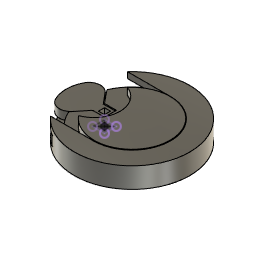
TotemMount (Autodesk Fusion 360 design; units mm, degrees)
Autodesk Fusion 360 part; units mm, degrees
sketch "Sketch1" plane through (0, 0, 0) normal (0, 0, 1) x (1, 0, 0)
  circle A0 centre (0, 0) radius 48
  dimension "d1" = 96
  constraint coincident A0.centre origin
  measures "d1" diameter of A0
extrude "Extrude1" add sketch "Sketch1" along normal blind 4 makes body 1
sketch "Sketch2" plane through (0, 0, 4) normal (0, 0, 1) x (-1, 0, 0)
  circle A0 centre (0, 0) radius 48
  line L0 (0, 0) -> (18, 0)
  line L1 (18, -4.925) -> (18, 4.925)
  line L2 (18, -4.925) -> (27.85, -4.925)
  line L3 (27.85, -4.925) -> (27.85, 4.925)
  line L4 (27.85, 4.925) -> (18, 4.925)
  circle A1 centre (0, 0) radius 40
  line L5 (0, -40) -> (50, -40)
  line L6 (0, 40) -> (50, 40)
  dimension "d4" = 18
  dimension "d5" = 9.85
  dimension "d6" = 8
  constraint coincident A0.centre L0.start
  constraint horizontal L0
  constraint vertical L1
  constraint midpoint L0.end L1
  constraint perpendicular L1 L2
  constraint equal L1 L2
  constraint perpendicular L2 L3
  constraint perpendicular L3 L4
  constraint concentric A0 A1
  constraint coincident A1 L5.start
  constraint tangent A1 L5
  constraint horizontal L5
  constraint coincident A1 L6.start
  constraint tangent A1 L6
  constraint horizontal L6
  measures "d4" distance of A0.centre L0.end
  measures "d5" distance of L1.start L2.end
  measures "d6" distance of A0 A1
extrude "Extrude2" cut sketch "Sketch2" against normal blind 30 contours L1 L2 L3 L4 bodies 1
extrude "Extrude3" add sketch "Sketch2" along normal blind 8 contours A0 A1 L5 L6 picked at (2.0777, 45.1772) bodies 1
sketch "Sketch3" plane through (0, 0, 12) normal (0, 0, 1) x (-1, 0, 0)
  arc A0 (0, 40) -> (0, -40) centre (0, 0) ccw
  line L0 (0, 40) -> (26.533, 40)
  arc A1 (26.533, 40) -> (26.533, -40) centre (0, 0) ccw
  line L1 (26.533, -40) -> (0, -40)
  circle A2 centre (0, 0) radius 32
  circle A3 centre (0, 0) radius 40
  line L2 (0, -32) -> (50, -32)
  line L3 (0, 32) -> (50.0906, 32)
  circle A4 centre (0, 0) radius 48
  circle A5 centre (0, 0) radius 48
  dimension "d11" = 8
  constraint coincident A0.centre A1.centre
  constraint coincident A2 L2.start
  constraint horizontal L2
  constraint coincident A2 L3.start
  constraint horizontal L3
  constraint collinear A0.start A0.end L2.start
  constraint collinear A0.start L2.start L3.start
  constraint concentric A2 A4
  constraint equal A4 A5
  measures "d11" distance of A2 A3
extrude "Extrude4" add sketch "Sketch3" along normal blind 5 contours A0 A2 A3 L2 L3 | A0 L0 A1 L1 A3 A4 A5 | L0 A3 L3 A4 A5 | L1 A3 L2 A4 A5 bodies 1
sketch "Sketch4" plane through (0, 0, 4) normal (0, 0, 1) x (-1, 0, 0)
  circle A0 centre (0, 0) radius 39.8
  circle A1 centre (0, 0) radius 40
  dimension "d14" = 0.2
  constraint coincident A0.centre A1.centre
  measures "d14" distance of A0 A1
extrude "Extrude5" add sketch "Sketch2" along normal blind 7.6 separate body contours A1 makes body 2
sketch "Sketch5" plane through (0, 0, 11.6) normal (0, 0, 1) x (-1, 0, 0)
  line L0 (27.85, -4.925) -> (18, -4.925)
  line L1 (18, -4.925) -> (18, 4.925)
  line L2 (18, 4.925) -> (27.85, 4.925)
  line L3 (27.85, 4.925) -> (27.85, -4.925)
  circle A0 centre (0, 0) radius 31.6
  arc A1 (0, 32) -> (0, -32) centre (0, 0) ccw
  circle A2 centre (31.6, 0) radius 21.6
  circle A3 centre (0, 0) radius 40
  dimension "d17" = 0.4
  dimension "d18" = 43.2
  constraint coincident A0 A2.centre
  measures "d17" distance of A0 A1
  measures "d18" diameter of A2
extrude "Extrude6" add sketch "Sketch5" along normal blind 5.7 contours A0 A2 picked at (-17.657, 0.5171) bodies 2
sketch "Sketch6" plane through (0, 0, 11.6) normal (0, 0, 1) x (-1, 0, 0)
  arc A0 (24.2177, 20.2993) -> (24.2177, -20.2993) centre (31.6, 0) ccw
  arc A1 (24.2177, 20.2993) -> (24.2177, -20.2993) centre (0, 0) ccw
  line L0 (27.85, -4.925) -> (18, -4.925)
  line L1 (18, -4.925) -> (18, 4.925)
  line L2 (18, 4.925) -> (27.85, 4.925)
  line L3 (27.85, 4.925) -> (27.85, -4.925)
  line L4 (27.85, -4.925) -> (36.7179, -15.868)
  line L5 (27.85, 4.925) -> (36.7179, 15.868)
  circle A2 centre (0, 0) radius 40
  constraint coincident L0.start L3.end
  constraint coincident L4.end A2
  constraint coincident L2.end L3.start
  constraint coincident L5.end A2
extrude "Extrude8" cut sketch "Sketch6" against normal blind 10 contours L3 L4 L5 A2 bodies 2
sketch "Sketch7" plane through (0, 0, 0) normal (0, 0, 1) x (1, 0, 0)
  line L0 (-27.55, 4.625) -> (-18.3, 4.625)
  line L1 (-18.3, 4.625) -> (-18.3, -4.625)
  line L2 (-18.3, -4.625) -> (-27.55, -4.625)
  line L3 (-27.55, -4.625) -> (-27.55, 4.625)
  line L4 (-27.55, 4.625) -> (-18.3, -4.625) construction
  line L5 (-18.3, 4.625) -> (-27.55, -4.625) construction
  line L6 (-18, 4.925) -> (-27.85, 4.925)
  line L7 (-27.85, -4.925) -> (-18, -4.925)
  line L8 (-18, 4.925) -> (-18, -4.925)
  line L9 (-25.425, 2.5) -> (-20.425, 2.5)
  line L10 (-20.425, 2.5) -> (-20.425, -2.5)
  line L11 (-20.425, -2.5) -> (-25.425, -2.5)
  line L12 (-25.425, -2.5) -> (-25.425, 2.5)
  line L13 (-25.425, 2.5) -> (-20.425, -2.5) construction
  line L14 (-20.425, 2.5) -> (-25.425, -2.5) construction
  point P0 (-22.925, 0)
  point P1 (-22.925, 0)
  dimension "d25" = 0.3
  dimension "d26" = 0.3
  dimension "d27" = 0.3
  dimension "d28" = 5
  dimension "d29" = 5
  constraint horizontal L0
  constraint perpendicular L0 L1
  constraint parallel L0 L2
  constraint parallel L1 L3
  constraint coincident L4 P1
  constraint coincident L5 P1
  constraint equal L0 L1
  constraint horizontal L9
  constraint perpendicular L9 L10
  constraint parallel L9 L11
  constraint parallel L10 L12
  constraint coincident L13 P1
  constraint coincident L14 P1
  constraint coincident P1 P0
  measures "d25" distance of L0 L6
  measures "d26" distance of L2 L7
  measures "d27" distance of L1 L8
  measures "d28" distance of L10.end L11.end
  measures "d29" distance of L9.end L10.end
extrude "Extrude9" add sketch "Sketch7" along normal blind 0.48 separate body contours L0 L1 L2 L3 | L9 L10 L11 L12 makes body 3
extrude "Extrude10" add sketch "Sketch7" along normal blind 11 bodies 3
sketch "Sketch8" plane through (-27.55, 0, 0) normal (-1, 0, 0) x (0, -1, 0)
  line L0 (-4.625, 0) -> (4.625, 0)
  line L1 (4.625, 0) -> (4.625, 11)
  line L2 (4.625, 11) -> (-4.625, 11)
  line L3 (-4.625, 11) -> (-4.625, 0)
  line L4 (-4.625, 11) -> (4.625, 11)
  line L5 (4.625, 11) -> (4.625, 4.1948)
  line L6 (4.625, 4.1948) -> (-4.625, 4.1948)
  line L7 (-4.625, 4.1948) -> (-4.625, 11)
  dimension "d34" = 6.8052
  constraint horizontal L4
  constraint vertical L5
  constraint horizontal L6
  constraint vertical L7
  constraint coincident L1 L5.end
  constraint coincident L2.end L3.start
  measures "d34" distance of L2.end L6.end
extrude "Extrude11" add sketch "Sketch8" along normal blind 18 contours L1 L2 L3 L4 L5 L6 L7 bodies 3
sketch "Sketch9" plane through (0, 0, 11) normal (0, 0, 1) x (-1, 0, 0)
  line L0 (20.425, 2.5) -> (25.425, 2.5)
  line L1 (25.425, 2.5) -> (25.425, -2.5)
  line L2 (25.425, -2.5) -> (20.425, -2.5)
  line L3 (20.425, -2.5) -> (20.425, 2.5)
  line L4 (45.55, 4.625) -> (18.3, 4.625)
  line L5 (18.3, 4.625) -> (18.3, -4.625)
  line L6 (18.3, -4.625) -> (45.55, -4.625)
  line L7 (45.55, -4.625) -> (45.55, 4.625)
  line L8 (28.5205, -4.625) -> (42.958, -21.8309)
  line L9 (28.5205, -4.625) -> (42.5512, -4.625) construction
  line L10 (28.5205, -4.625) -> (28.5205, 4.625)
  line L11 (28.5205, 4.625) -> (42.958, 21.8309)
  circle A0 centre (28.5205, 0) radius 26.173
  dimension "d37" = 50
  dimension "d38" = 140
  constraint horizontal L9
  constraint coincident L6 L8.start
  constraint coincident L4 L10.end
  constraint perpendicular L4 L10
  constraint midpoint L10 A0.centre
  constraint coincident L8.end A0
  constraint coincident L11.end A0
  measures "d37" angle of L8 L9
  measures "d38" angle of L10 L11
extrude "Extrude12" add sketch "Sketch9" against normal blind 6.8 contours L4 L6 L7 L10 | L4 L6 L7 L8 L11 A0 bodies 3
fillet "Fillet1" radius 9.5 2 edges at (-42.958, -21.8309, 7.6) (-42.958, 21.8309, 7.6) on bodies 3
